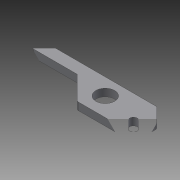
# Autodesk Inventor part: Air2D_Hinge_Sideplate
Saved by Autodesk Inventor 2014 (Build 180170000, 170)
## iProperties
Created: 2014-09-30
Part Number: Air2D_Hinge_Sideplate
Material: Generic
Document SubType Name: Modeling
Designer: ThatOtherGuy
Density: 1 g/cm^3
Appearance: Default
Author: ThatOtherGuy
Autodesk Inventor part; units mm, degrees
ref_plane "YZ Plane" through (0, 0, 0) normal (1, 0, 0) x (0, 1, 0)
ref_plane "XZ Plane" through (0, 0, 0) normal (0, 1, 0) x (-1, 0, 0)
ref_plane "XY Plane" through (0, 0, 0) normal (0, 0, 1) x (1, 0, 0)
sketch "Sketch1" plane through (0, 0, 0) normal (0, 0, 1) x (1, 0, 0)
  line L0 (30, 0) -> (54, 0)
  line L1 (54, 0) -> (54, 10)
  circle A0 centre (49, 5) radius 1.6
  circle A1 centre (34, 8) radius 4
  line L2 (49, 15) -> (54, 10)
  line L3 (30, 0) -> (20, 10)
  line L4 (0, 15) -> (0, 10)
  line L5 (0, 10) -> (0, 12.5)
  line L6 (20, 10) -> (0, 10)
  line L7 (0, 15) -> (0, 17)
  line L8 (0, 17) -> (5, 17)
  line L9 (5, 17) -> (5, 15)
  line L10 (30, 15) -> (0, 15)
  line L11 (49, 15) -> (30, 15)
  line L12 (30, 15) -> (30, 15)
  point P0 (0, 0)
  dimension "d0" = 3.2
  dimension "d1" = 8
  dimension "d3" = 15
  dimension "d4" = 5
  dimension "d5" = 5
  dimension "d10" = 8
  dimension "d13" = 10
  dimension "d29" = 5
  dimension "d30" = 2
  dimension "d33" = 15
  dimension "d34" = 45
  dimension "d37" = 20
  dimension "d38" = 5
  dimension "d42" = 10
  dimension "d44" = 34
  dimension "d45" = 19
  dimension "d46" = 0
  constraints: 26 end point, 6 perpendicular, 3 parallel, 2 centre point, 2 point on line, 1 collinear, 1 horizontal, 1 horizontal alignment, 1 midpoint, 1 vertical alignment
  measures "d0" diameter of A0
  measures "d1" diameter of A1
  measures "d3" horizontal distance of A0.centre A1.centre
  measures "d4" distance from line of L0 A0.centre
  measures "d5" distance from line of A0.centre L1
  measures "d10" distance from line of L0 A1.centre
  measures "d13" distance of L0.end L1.end
  measures "d29" distance of L7.end L8.end
  measures "d30" distance of L8.end L9.end
  measures "d33" distance between parallel lines of L0 L11
  measures "d34" angle of L1 L2
  measures "d37" distance of L3.end L4.end
  measures "d38" distance of L4.start L4.end
  measures "d42" distance between parallel lines of L6 L0
  measures "d44" distance from line of L1 L3.end
  measures "d45" distance of L2.start L11.end
  measures "d46" distance between parallel lines of L4 L7
extrude "Extrusion1" add sketch "Sketch1" along normal blind 3.175
fillet "Fillet1" radius 1.5875 4 edges at (54, 10, 1.5875) (0, 10, 1.5875) (30, 0, 1.5875) (49, 15, 1.5875)
fillet "Fillet1" radius 5 1 edges at (54, 0, 1.5875)
equation "\"d7\" = THICKA"
equation "\"THICKA\" = 3.175"
equation "\"THICKB\" = 6.731"
equation "\"THICKC\" = 12.7"
equation "\"BALLDIA\" = 12"
equation "\"MAGDIA\" = 9.5"
body "Solid1"
